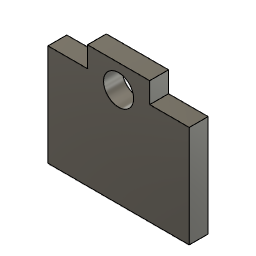
CP-BO PCF8574 locker v2 (Autodesk Fusion 360 design; units mm, degrees)
Autodesk Fusion 360 part; units mm, degrees
sketch "Esquisse1" plane through (0, 0, 0) normal (0, 0, 1) x (1, 0, 0)
  line L0 (0, 0) -> (15, 0)
  line L1 (15, 0) -> (15, 13)
  line L2 (15, 13) -> (0, 13)
  line L3 (0, 13) -> (0, 0)
  line L4 (0, 13) -> (4.2, 13)
  line L5 (4.2, 13) -> (4.2, 10.8)
  line L6 (4.2, 10.8) -> (0, 10.8)
  line L7 (0, 10.8) -> (0, 13)
  line L8 (15, 13) -> (10.8, 13)
  line L9 (10.8, 13) -> (10.8, 10.8)
  line L10 (10.8, 10.8) -> (15, 10.8)
  line L11 (15, 10.8) -> (15, 13)
  line L12 (0, 8) -> (15, 8) construction
  line L13 (7.5, 8) -> (7.5, 13) construction
  circle A0 centre (7.5, 10.5) radius 1.6
  dimension "d1" = 15
  dimension "d2" = 13
  dimension "d3" = 4.2
  dimension "d4" = 2.2
  dimension "d5" = 4.2
  dimension "d6" = 2.2
  dimension "d9" = 5
  dimension "d10" = 3.2
  constraint horizontal L0
  constraint vertical L1
  constraint horizontal L2
  constraint vertical L3
  constraint coincident L0.start L3.end
  constraint horizontal L4
  constraint vertical L5
  constraint horizontal L6
  constraint vertical L7
  constraint horizontal L8
  constraint vertical L9
  constraint horizontal L10
  constraint vertical L11
  constraint coincident L3 L12.start
  constraint coincident L1 L12.end
  constraint perpendicular L1 L12
  constraint midpoint L12 L13.start
  constraint midpoint L2 L13.end
  constraint midpoint L13 A0.centre
  measures "d1" distance of L0.start L0.end
  measures "d2" distance of L0.start L2.end
  measures "d3" distance of L2.end L4.end
  measures "d4" distance of L2.end L6.end
  measures "d5" distance of L1.end L8.end
  measures "d6" distance of L1.end L10.end
  measures "d9" distance of L2 L12
  measures "d10" diameter of A0
extrude "Extrusion1" add sketch "Esquisse1" along normal blind 2 contours L0 L1 L2 L3 L5 L6 L9 L10
